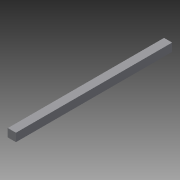
# Autodesk Inventor part: TemporaryBlock
Saved by Autodesk Inventor 2013 (Build 170138000, 138)
## iProperties
Created: 2014-01-09
Part Number: TemporaryBlock
Material: Generic
Document SubType Name: Modeling
Designer: 215152
Density: 1 g/cm^3
Author: 215152
Autodesk Inventor part; units mm, degrees
ref_plane "YZ Plane" through (0, 0, 0) normal (1, 0, 0) x (0, 1, 0)
ref_plane "XZ Plane" through (0, 0, 0) normal (0, 1, 0) x (-1, 0, 0)
ref_plane "XY Plane" through (0, 0, 0) normal (0, 0, 1) x (1, 0, 0)
sketch "Sketch1" plane through (0, 0, 0) normal (0, 0, 1) x (1, 0, 0)
  line L0 (0, 0) -> (-647.7, 0)
  line L1 (-647.7, 0) -> (-644.525, 0)
  line L2 (-644.525, 0) -> (-644.525, -3.175)
  line L3 (-644.525, -3.175) -> (-647.7, -3.175)
  line L4 (-647.7, -3.175) -> (-647.7, 0)
  dimension "d0" = 647.7
  dimension "d1" = 3.175
  dimension "d2" = 3.175
  constraints: 10 end point, 2 horizontal, 2 parallel, 1 perpendicular
  measures "d0" distance of L0.start L0.end
  measures "d1" distance of L2.end L3.end
  measures "d2" distance of L1.end L2.end
extrude "Extrusion1" add sketch "Sketch1" along normal blind 61.0398
body "Solid1"
